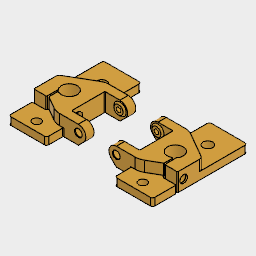
XY_Idler_Mount_1.0_F01 (Autodesk Fusion 360 design; units mm, degrees)
Autodesk Fusion 360 part; units mm, degrees
sketch "スケッチ1" plane through (0, 0, 0) normal (0, 0, 1) x (1, 0, 0)
  line L0 (-12.5, 35) -> (12.5, 35)
  line L1 (12.5, 35) -> (12.5, -27.5)
  line L2 (12.5, -27.5) -> (-12.5, -27.5)
  line L3 (-12.5, -27.5) -> (-12.5, 35)
  line L4 (-12.5, 35) -> (12.5, -27.5) construction
  line L5 (12.5, 35) -> (-12.5, -27.5) construction
  circle A0 centre (0, 0) radius 5.2
  circle A1 centre (0, -21.5) radius 2.7
  circle A2 centre (0, 21.5) radius 3.2
  line L6 (-12.5, -12) -> (-3, -12)
  line L7 (-3, -12) -> (-3, -4.2474)
  line L8 (-12.5, -11) -> (-4, -11)
  line L9 (-4, -11) -> (-4, -3.3226)
  line L10 (-12.5, 5) -> (7.4186, 16.5)
  line L11 (7.4186, 16.5) -> (27.5, 16.5)
  line L12 (27.5, 16.5) -> (27.5, 11)
  line L13 (27.5, 11) -> (12.5, 11)
  line L14 (-12.5, -5) -> (7.4186, -16.5)
  line L15 (7.4186, -16.5) -> (27.5, -16.5)
  line L16 (27.5, -16.5) -> (27.5, -11)
  line L17 (27.5, -11) -> (12.5, -11)
  circle A3 centre (0, 21.5) radius 4.75 construction
  point P0 (0, 3.75)
  dimension "d1" = 62.5
  dimension "d2" = 25
  dimension "d3" = 10.4
  dimension "d4" = 27.5
  dimension "d5" = 5.4
  dimension "d6" = 6.4
  dimension "d7" = 13.5
  dimension "d8" = 6
  dimension "d9" = 15.5
  dimension "d10" = 1
  dimension "d11" = 1
  dimension "d12" = 8.5
  dimension "d13" = 60
  dimension "d14" = 5
  dimension "d15" = 5
  dimension "d16" = 60
  dimension "d17" = 16.5
  dimension "d18" = 16.5
  dimension "d19" = 5.5
  dimension "d20" = 5.5
  dimension "d21" = 15
  dimension "d22" = 15
  dimension "d77" = 9.5
  measures "d1" distance of L0.end L1.end
  measures "d2" distance of L1.end L2.end
  measures "d3" diameter of A0
  measures "d4" distance of A0.centre L2
  measures "d5" diameter of A1
  measures "d6" diameter of A2
  measures "d7" distance of L0 A2.centre
  measures "d8" distance of L2 A1.centre
  measures "d9" distance of L2 L6
  measures "d10" distance of L6 L8
  measures "d11" distance of L7 L9
  measures "d12" distance of L3 L9
  measures "d13" angle of L3 L10
  measures "d14" distance of A0.centre L10.start
  measures "d15" distance of A0.centre L14.start
  measures "d16" angle of L3 L14
  measures "d17" distance of A0.centre L11
  measures "d18" distance of A0.centre L15
  measures "d19" distance of L15 L17
  measures "d20" distance of L11 L13
  measures "d21" distance of L1 L12
  measures "d22" distance of L1 L16
  measures "d77" diameter of A3
extrude "押し出し1" add sketch "スケッチ1" along normal blind 5 contours L0 L1 L3 L10 L11 | L1 L3 A0 L7 L9 L10 L11 L14 L15 | L3 L8 L9 L14 | L1 L2 L3 L6 L7 L14 L15 makes body 1
extrude "押し出し2" add sketch "スケッチ1" along normal blind 12 contours L1 L3 A0 L7 L9 L10 L11 L14 L15 | L1 L11 L12 L13 | L3 L8 L9 L14 | L1 L15 L16 L17 bodies 1
fillet "フィレット1" radius 1.5 4 edges at (12.5, 35, 2.5) (-12.5, 35, 2.5) (-12.5, -27.5, 2.5) (12.5, -27.5, 2.5) on bodies 1
fillet "フィレット2" radius 10 2 edges at (7.4186, 16.5, 8.5) (7.4186, -16.5, 8.5) on bodies 1
fillet "フィレット3" radius 2.5 1 edges at (-12.5, 5, 8.5) on bodies 1
fillet "フィレット4" radius 0.5 6 edges at (-3, -4.2474, 6) (-4, -3.3226, 6) (-4, -11, 6) (-12.5, -11, 6) (-12.5, -12, 2.5) (-3, -10.4848, 8.5) on bodies 1
fillet "フィレット5" radius 1.5 1 edges at (-3, -12, 2.5) on bodies 1
fillet "フィレット6" radius 0.5 4 edges at (12.5, 16.5, 2.5) (12.5, -11, 6) (12.5, 11, 6) (12.5, -16.5, 2.5) on bodies 1
sketch "スケッチ2" plane through (0, 11, 0) normal (0, -1, 0) x (1, 0, 0)
  line L0 (13, 12) -> (13, 0)
  line L1 (13, 0) -> (27.5, 0)
  line L2 (27.5, 0) -> (27.5, 12)
  line L3 (27.5, 12) -> (13, 12)
  circle A0 centre (22.5, 7) radius 4
  line L4 (10.0981, 12) -> (27.5, 12)
  line L5 (27.5, 0) -> (27.5, 12)
  dimension "d33" = 8
  dimension "d34" = 5
  dimension "d35" = 5
  measures "d33" diameter of A0
  measures "d34" distance of A0.centre L4
  measures "d35" distance of A0.centre L5
extrude "押し出し3" add sketch "スケッチ2" along normal blind 1 draft -45 contours A0 bodies 1
sketch "スケッチ3" plane through (0, 10, 0) normal (0, -1, 0) x (1, 0, 0)
  circle A0 centre (22.5, 7) radius 3
  circle A1 centre (22.5, 7) radius 1.5
  dimension "d38" = 3
  measures "d38" diameter of A1
extrude "押し出し4" cut sketch "スケッチ3" against normal blind 8 contours A1 bodies 1
sketch "スケッチ4" plane through (0, -11, 0) normal (0, 1, 0) x (-1, 0, 0)
  line L0 (-13, 0) -> (-13, 12)
  line L1 (-13, 12) -> (-27.5, 12)
  line L2 (-27.5, 12) -> (-27.5, 0)
  line L3 (-27.5, 0) -> (-13, 0)
  circle A0 centre (-22.5, 7) radius 4
  dimension "d41" = 8
  dimension "d42" = 5
  dimension "d43" = 5
  measures "d41" diameter of A0
  measures "d42" distance of L1 A0.centre
  measures "d43" distance of L2 A0.centre
extrude "押し出し5" add sketch "スケッチ4" along normal blind 1 draft -45 contours A0 bodies 1
sketch "スケッチ5" plane through (0, -10, 0) normal (0, 1, 0) x (-1, 0, 0)
  circle A0 centre (-22.5, 7) radius 3
  circle A1 centre (-22.5, 7) radius 1.5
  dimension "d46" = 3
  measures "d46" diameter of A1
extrude "押し出し6" cut sketch "スケッチ5" against normal blind 8 contours A1 bodies 1
sketch "スケッチ6" plane through (0, 16.5, 0) normal (0, 1, 0) x (-1, 0, 0)
  circle A0 centre (-22.5, 7) radius 1.5
  line L0 (-13, 0) -> (-13, 5)
  line L1 (-13, 5) -> (-10.0981, 5)
  line L2 (-10.0981, 5) -> (-10.0981, 12)
  line L3 (-10.0981, 12) -> (-27.5, 12)
  line L4 (-27.5, 12) -> (-27.5, 0)
  line L5 (-27.5, 0) -> (-13, 0)
  circle A1 centre (-22.5, 7) radius 3.1
  dimension "d49" = 6.2
  measures "d49" diameter of A1
extrude "押し出し7" cut sketch "スケッチ6" against normal blind 1.5 contours A1 bodies 1
sketch "スケッチ7" plane through (0, -16.5, 0) normal (0, -1, 0) x (1, 0, 0)
  circle A0 centre (22.5, 7) radius 1.5
  line L0 (13, 5) -> (13, 0)
  line L1 (13, 0) -> (27.5, 0)
  line L2 (27.5, 0) -> (27.5, 12)
  line L3 (27.5, 12) -> (10.0981, 12)
  line L4 (10.0981, 12) -> (10.0981, 5)
  line L5 (10.0981, 5) -> (13, 5)
  circle A1 centre (22.5, 7) radius 2.5
  circle A2 centre (22.5, 7) radius 2.35
  dimension "d52" = 5
  dimension "d53" = 4.7
  measures "d52" diameter of A1
  measures "d53" diameter of A2
extrude "押し出し8" cut sketch "スケッチ7" against normal blind 5 contours A2 bodies 1
extrude "押し出し9" cut sketch "スケッチ7" against normal blind 0.5 contours A1 bodies 1
fillet "フィレット7" radius 5 2 edges at (27.5, 13.75, 12) (27.5, -13.75, 12) on bodies 1
chamfer "面取り1" distance 5 angle 45 2 edges at (27.5, 13.75, 0) (27.5, -13.75, 0) on bodies 1
fillet "フィレット8" radius 5 2 edges at (27.5, -13.75, 5) (27.5, 13.75, 5) on bodies 1
sketch "スケッチ8" plane through (12.5, 0, 0) normal (1, 0, 0) x (0, 1, 0)
  line L0 (10.5, 0) -> (10.5, 12)
  line L1 (10.5, 12) -> (-10.5, 12)
  line L2 (-10.5, 12) -> (-10.5, 0)
  line L3 (-10.5, 0) -> (10.5, 0)
  circle A0 centre (-7, 6) radius 1.75
  circle A1 centre (-7, 6) radius 3.25
  dimension "d61" = 3.5
  dimension "d62" = 7
  dimension "d63" = 6
  dimension "d64" = 6.5
  measures "d61" diameter of A0
  measures "d62" distance of origin A0.centre
  measures "d63" distance of L3 A0.centre
  measures "d64" diameter of A1
extrude "押し出し10" cut sketch "スケッチ8" against normal blind 30 contours A0 bodies 1
extrude "押し出し11" cut sketch "スケッチ8" against normal blind 3 contours A1 bodies 1
sketch "スケッチ9" plane through (-12.5, 0, 0) normal (-1, 0, 0) x (0, -1, 0)
  circle A0 centre (7, 6) radius 1.75
  line L0 (10.5, 0) -> (10.5, 12)
  line L1 (10.5, 12) -> (-3.5566, 12)
  line L2 (-3.5566, 12) -> (-3.5566, 5)
  line L3 (-3.5566, 5) -> (-33.5, 5)
  line L4 (-33.5, 5) -> (-33.5, 0)
  line L5 (-33.5, 0) -> (10.5, 0)
  circle A1 centre (7, 6) radius 2.5
  circle A2 centre (7, 6) radius 2.35
  dimension "d69" = 5
  dimension "d70" = 4.7
  measures "d69" diameter of A1
  measures "d70" diameter of A2
extrude "押し出し12" cut sketch "スケッチ9" against normal blind 5 contours A2 bodies 1
extrude "押し出し13" cut sketch "スケッチ9" against normal blind 1 contours A1 bodies 1
ref_plane "作業平面1" through (35, 0, 0) normal (1, 0, 0) x (0, 1, 0)
mirror "ミラー1" about plane through (35, 0, 0) normal (1, 0, 0) of bodies 1 makes body 2
